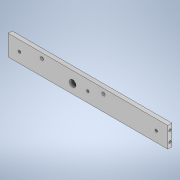
# Autodesk Inventor part: Frente
Saved by Autodesk Inventor 2020 (Build 240168000, 168)
## iProperties
Created: 2020-04-28
Part Number: Frente
Material: Aluminio 6061
Document SubType Name: Modeling
Designer: Dante
Density: 2.7 g/cm^3
Appearance: Aluminum - Dark
Mass: 802.916 g
Surface Area: 634.044 cm^2
Volume: 297.376 cm^3
Author: Dante
Autodesk Inventor part; units mm, degrees
ref_plane "YZ Plane" through (0, 0, 0) normal (1, 0, 0) x (0, 1, 0)
ref_plane "XZ Plane" through (0, 0, 0) normal (0, 1, 0) x (-1, 0, 0)
ref_plane "XY Plane" through (0, 0, 0) normal (0, 0, 1) x (1, 0, 0)
sketch "Sketch1" plane through (0, 0, 0) normal (0, 0, 1) x (1, 0, 0)
  line L0 (-86, 40) -> (-86, 90)
  line L1 (-86, 90) -> (304, 90)
  line L2 (304, 90) -> (304, 40)
  circle A0 centre (72, 63) radius 8
  circle A1 centre (147, 78) radius 4
  circle A2 centre (-3, 78) radius 4
  line L3 (-86, 40) -> (304, 40)
  circle A3 centre (-58, 65) radius 3
  circle A4 centre (276, 65) radius 3
  circle A5 centre (109, 65) radius 3
  dimension "d1" = 390
  dimension "d2" = 16
  dimension "d6" = 8
  dimension "d7" = 8
  dimension "d8" = 15
  dimension "d13" = 75
  dimension "d14" = 75
  dimension "d27" = 15
  dimension "d38" = 50
  dimension "d58" = 27
  dimension "d68" = 232
  dimension "d69" = 6
  dimension "d70" = 25
  dimension "d71" = 28
  dimension "d72" = 6
  dimension "d73" = 25
  dimension "d74" = 28
  dimension "d75" = 6
  dimension "d76" = 25
  dimension "d77" = 195
  constraints: 8 end point, 6 centre point, 2 vertical, 1 horizontal, 1 perpendicular
  measures "d1" distance of L0.end L1.end
  measures "d2" diameter of A0
  measures "d6" diameter of A1
  measures "d7" diameter of A2
  measures "d8" vertical distance of A1.centre A0.centre
  measures "d13" horizontal distance of A0.centre A1.centre
  measures "d14" horizontal distance of A2.centre A0.centre
  measures "d27" vertical distance of A2.centre A0.centre
  measures "d38" distance of L0.start L0.end
  measures "d58" distance from line of L1 A0.centre
  measures "d68" distance from line of A0.centre L2
  measures "d69" diameter of A3
  measures "d70" distance from line of L1 A3.centre
  measures "d71" distance from line of L0 A3.centre
  measures "d72" diameter of A4
  measures "d73" distance from line of L1 A4.centre
  measures "d74" distance from line of L2 A4.centre
  measures "d75" diameter of A5
  measures "d76" distance from line of L1 A5.centre
  measures "d77" distance from line of L2 A5.centre
extrude "Extrusión3" add sketch "Sketch1" along normal blind 10
sketch "Boceto3" plane through (304, 40, 0) normal (1, 0, 0) x (0, 0, -1)
  line L0 (-10, 0) -> (-10, 50) projected
  line L1 (-10, 50) -> (-5, 50)
  line L2 (0, 50) -> (-10, 50) projected
  line L3 (0, 0) -> (0, 50) projected
  line L4 (-5, 0) -> (-5, 12.5)
  line L5 (-5, 50) -> (-5, 37.5)
  circle A0 centre (-5, 37.5) radius 3
  circle A1 centre (-5, 12.5) radius 3
  point P0 (0, -40)
  dimension "d42" = 5
  dimension "d43" = 50
  dimension "d44" = 12.5
  dimension "d45" = 12.5
  dimension "d46" = 6
  dimension "d47" = 6
  constraints: 6 end point, 2 centre point, 2 coincident, 1 midpoint
  measures "d42" distance of L0.end L1.end
  measures "d43" distance of L1.end L4.start
  measures "d44" distance of L4.start L4.end
  measures "d45" distance of L1.end L5.end
  measures "d46" diameter of A0
  measures "d47" diameter of A1
extrude "Extrusión4" cut sketch "Boceto3" against normal blind 15
sketch "Boceto4" plane through (-86, 40, 0) normal (-1, 0, 0) x (0, 0, 1)
  line L0 (10, 0) -> (10, 50) projected
  line L1 (10, 50) -> (5, 50)
  line L2 (0, 50) -> (10, 50) projected
  line L3 (5, 50) -> (5, 0)
  line L4 (5, 0) -> (5, 12.5)
  line L5 (5, 50) -> (5, 37.5)
  circle A0 centre (5, 12.5) radius 3
  circle A1 centre (5, 37.5) radius 3
  point P0 (0, -40)
  dimension "d50" = 5
  dimension "d51" = 50
  dimension "d52" = 12.5
  dimension "d53" = 12.5
  constraints: 8 end point, 2 centre point, 2 coincident, 2 point on line, 1 midpoint, 1 perpendicular
  measures "d50" distance of L0.end L1.end
  measures "d51" distance of L1.end L3.end
  measures "d52" distance of L3.end L4.end
  measures "d53" distance of L1.end L5.end
extrude "Extrusión5" cut sketch "Boceto4" against normal blind 15
thread "Rosca1" size "M6x1" class "6H" standard "ISO Metric profile" length 430
thread "Rosca2" size "M6x1" class "6H" standard "ISO Metric profile" length 430
thread "Rosca3" size "M6x1" class "6H" standard "ISO Metric profile" length 430
thread "Rosca4" size "M6x1" class "6H" standard "ISO Metric profile" length 430
thread "Rosca5" size "M6x1" class "6H" standard "ISO Metric profile" length 100
thread "Rosca6" size "M6x1" class "6H" standard "ISO Metric profile" length 100
thread "Rosca7" size "M6x1" class "6H" standard "ISO Metric profile" length 100
equation "\"d73\" = d70"
equation "\"d74\" = d71"
equation "\"d76\" = d70"
